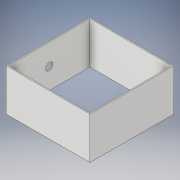
# Autodesk Inventor part: MAN_BASIS_PRIMARY_STRUCTURE
Saved by Autodesk Inventor 2019 (Build 230136000, 136)
## iProperties
Created: 2021-03-07
Part Number: MAN_BASIS_PRIMARY_STRUCTURE
Material: ABS Plastic
Document SubType Name: Modeling
Designer: DOMEK
Density: 1.06 g/cm^3
Appearance: Smooth - White
Author: DOMEK
Autodesk Inventor part; units mm, degrees
ref_plane "YZ Plane" through (0, 0, 0) normal (1, 0, 0) x (0, 1, 0)
ref_plane "XZ Plane" through (0, 0, 0) normal (0, 1, 0) x (-1, 0, 0)
ref_plane "XY Plane" through (0, 0, 0) normal (0, 0, 1) x (1, 0, 0)
sketch "Sketch12" plane through (0, 0, 0) normal (0, 1, 0) x (-1, 0, 0)
  line L0 (0, 0) -> (0, 40)
  line L1 (0, 40) -> (80, 40)
  line L2 (80, 40) -> (80, 0)
  line L3 (80, 0) -> (80, -40)
  line L4 (80, -40) -> (0, -40)
  line L5 (0, -40) -> (0, 0)
  dimension "d39" = 40
  dimension "d40" = 80
  dimension "d41" = 40
  constraints: 12 end point, 4 perpendicular, 2 point on line, 1 vertical
  measures "d39" distance of L0.start L0.end
  measures "d40" distance of L0.end L1.end
  measures "d41" distance of L2.end L3.end
extrude "Extrusion10" add sketch "Sketch12" along normal blind 40
shell "Shell2" thickness 1 removed faces 2 at (-26.6667, 40, -13.3333) at (-26.6667, 0, -13.3333)
sketch "Sketch13" plane through (-80, 0, -40) normal (-1, 0, 0) x (0, 0, 1)
  line L0 (0, 0) -> (80, 0) projected
  line L1 (80, 40) -> (0, 40) projected
  circle A0 centre (40, 20) radius 3.5
  point P0 (40, 0)
  dimension "d45" = 7
  constraints: 1 centre point
  measures "d45" diameter of A0
extrude "Extrusion11" cut sketch "Sketch13" against normal blind 1
body "Solid3"
